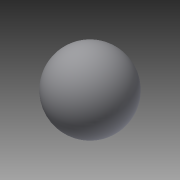
# Autodesk Inventor part: rueda loca bola
Saved by Autodesk Inventor 2015 (Build 190159000, 159)
## iProperties
Created: 2015-11-29
Part Number: rueda loca bola
Material: Genérico
Document SubType Name: Modeling
Designer: user
Density: 1 g/cm^3
Appearance: Valor por defecto
Author: user
Autodesk Inventor part; units mm, degrees
ref_plane "YZ Plane" through (0, 0, 0) normal (1, 0, 0) x (0, 1, 0)
ref_plane "XZ Plane" through (0, 0, 0) normal (0, 1, 0) x (-1, 0, 0)
ref_plane "XY Plane" through (0, 0, 0) normal (0, 0, 1) x (1, 0, 0)
sketch "Boceto1" plane through (0, 0, 0) normal (0, 1, 0) x (-1, 0, 0)
  arc A0 (4.25, 0) -> (-4.25, 0) centre (0, 0) ccw
  line L0 (4.25, 0) -> (-4.25, 0)
  dimension "d0" = 8.5
  constraints: 2 end point, 2 point on circle, 1 centre point, 1 coincident, 1 horizontal
  measures "d0" diameter of A0
revolve "Revolución1" add sketch "Boceto1" angle 360 about axis through (-4.25, 0, 0) along (1, 0, 0)
